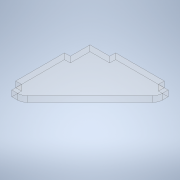
# Autodesk Inventor part: trackingCamAngleSupport
Saved by Autodesk Inventor 2020 (Build 240168000, 168)
## iProperties
Created: 2020-03-02
Part Number: trackingCamAngleSupport
Material: Polycarbonate, Clear
Document SubType Name: Modeling
Designer: n10208577
Density: 1.2 g/cm^3
Appearance: Polycarbonate - Clear
Author: n10208577
Autodesk Inventor part; units mm, degrees
ref_plane "YZ Plane" through (0, 0, 0) normal (1, 0, 0) x (0, 1, 0)
ref_plane "XZ Plane" through (0, 0, 0) normal (0, 1, 0) x (-1, 0, 0)
ref_plane "XY Plane" through (0, 0, 0) normal (0, 0, 1) x (1, 0, 0)
sketch "Sketch1" plane through (0, 0, 0) normal (0, 1, 0) x (-1, 0, 0)
  line L0 (39.5715, 34.4499) -> (39.5715, 9.4499)
  line L1 (39.5715, 34.4499) -> (36.5715, 34.4499)
  line L2 (39.5715, 9.4499) -> (36.5715, 9.4499)
  line L3 (36.5715, 9.4499) -> (36.5715, -0.6501)
  line L4 (36.5715, -0.6501) -> (26.4715, -0.6501)
  line L5 (26.4715, -3.6501) -> (1.4715, -3.6501)
  line L6 (26.4715, -3.6501) -> (26.4715, -0.6501)
  line L7 (1.4715, -3.6501) -> (1.4715, -0.6501)
  line L8 (36.5715, 34.4499) -> (36.5715, 39.4499)
  line L9 (1.4715, -0.6501) -> (-3.5285, -0.6501)
  line L10 (-3.5285, -0.6501) -> (-3.5285, 2.2788)
  line L11 (36.5715, 39.4499) -> (33.6426, 39.4499)
  arc A0 (33.6426, 39.4499) -> (30.1071, 37.9854) centre (33.6426, 34.4499) ccw
  line L12 (-2.064, 5.8143) -> (30.1071, 37.9854)
  arc A1 (-2.064, 5.8143) -> (-3.5285, 2.2788) centre (1.4715, 2.2788) ccw
  point P0 (0, 0)
  constraints: 26 end point, 4 point on circle, 2 centre point
extrude "Extrusion1" add sketch "Sketch1" along normal blind 3
body "Solid1"
